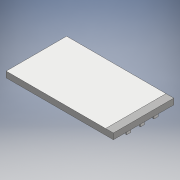
# Autodesk Inventor part: DISP BKL LED TB1012S
Saved by Autodesk Inventor 2018 (Build 220112000, 112)
## iProperties
Created: 2018-02-18
Part Number: DISP BKL LED TB1012S
Material: Generic
Document SubType Name: Modeling
Designer: danil
Density: 1 g/cm^3
Appearance: Default
Mass: 10.2861 g
Surface Area: 134.254 cm^2
Volume: 10.2861 cm^3
Author: danil
Autodesk Inventor part; units mm, degrees
ref_plane "YZ Plane" through (0, 0, 0) normal (1, 0, 0) x (0, 1, 0)
ref_plane "XZ Plane" through (0, 0, 0) normal (0, 1, 0) x (-1, 0, 0)
ref_plane "XY Plane" through (0, 0, 0) normal (0, 0, 1) x (1, 0, 0)
sketch "Sketch10" plane through (0, 0, 0) normal (0, 0, 1) x (1, 0, 0)
  line L0 (-27.5, -15.5) -> (27.5, -15.5)
  line L1 (27.5, -15.5) -> (27.5, 15.5)
  line L2 (27.5, 15.5) -> (-27.5, 15.5)
  line L3 (-27.5, 15.5) -> (-27.5, -15.5)
  line L4 (-27.5, -15.5) -> (27.5, 15.5) construction
  line L5 (27.5, -15.5) -> (-27.5, 15.5) construction
  point P0 (0, 0)
  dimension "d58" = 55
  dimension "d59" = 31
  constraints: 12 end point, 2 midpoint, 2 parallel, 1 horizontal, 1 perpendicular, 1 other
  measures "d58" distance of L2.end L1.end
  measures "d59" distance of L1.end L0.end
extrude "Extrusion9" add sketch "Sketch10" along normal blind 3
sketch "Sketch12" plane through (0, 0, 3) normal (0, 0, 1) x (1, 0, 0)
  line L0 (27.5, -15.5) -> (27.5, 15.5) projected
  line L1 (-27.5, -15.5) -> (27.5, -15.5) projected
  line L2 (27.5, 15.5) -> (23.5, 15.5)
  line L3 (23.5, 15.5) -> (23.5, -15.5)
  line L4 (23.5, -15.5) -> (27.5, -15.5)
  line L5 (27.5, -15.5) -> (27.5, 15.5)
  point P0 (0, 0)
  dimension "d72" = 4
  constraints: 8 end point, 2 parallel, 1 horizontal, 1 perpendicular, 1 point on line
  measures "d72" distance of L4.end L3.end
extrude "Extrusion11" add sketch "Sketch12" along normal blind 0.001
sketch "Sketch11" plane through (-12.75, 0, 0) normal (0, 0, -1) x (-1, 0, 0)
  line L0 (-39.65, -1.1) -> (-39.05, -1.1)
  line L1 (-39.05, -1.1) -> (-39.05, 1.1)
  line L2 (-39.05, 1.1) -> (-39.65, 1.1)
  line L3 (-39.65, 1.1) -> (-39.65, -1.1)
  line L4 (-40.25, -15.5) -> (-40.25, 15.5)
  line L5 (-40.25, -15.5) -> (-40.25, 15.5) projected
  point P0 (-39.65, 0)
  point P1 (-40.25, 0)
  point P2 (-40.25, 0)
  dimension "d64" = 0.6
  dimension "d65" = 2.2
  dimension "d63" = 0.6
  constraints: 10 end point, 3 midpoint, 2 horizontal alignment, 2 parallel, 1 collinear, 1 horizontal, 1 perpendicular
  measures "d64" distance of L2.end L1.end
  measures "d65" distance of L1.end L0.end
  measures "d63" distance between parallel lines of L4 L3
extrude "Extrusion10" add sketch "Sketch11" along normal blind 1.8 separate body
pattern_linear "Rectangular Pattern1" count 3 spacing 7 along (0, -1, 0) of "Extrusion10" first direction both ways yes bodies 2
body "Solid7"
body "Solid8"
